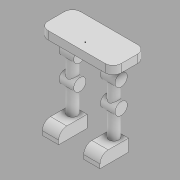
# Autodesk Inventor part: stick nodes
Saved by Autodesk Inventor 2021 (Build 250183000, 183)
## iProperties
Created: 2022-07-21
Part Number: stick nodes
Material: Generic
Document SubType Name: Modeling
Designer: Ahmed badghaish
Density: 1 g/cm^3
Appearance: Default
Author: Ahmed badghaish
Autodesk Inventor part; units mm, degrees
sketch "Sketch1" plane through (0, 0, 0) normal (0, 0, 1) x (1, 0, 0)
  line L0 (0, 0) -> (0, 200)
  line L1 (0, 0) -> (-50, 0)
  line L2 (0, 0) -> (50, 0)
  line L3 (-15.3846, 0) -> (-35.3846, 0)
  line L4 (-35.3846, 0) -> (-35.3846, 15)
  line L5 (-35.3846, 15) -> (-15.3846, 15)
  line L6 (-15.3846, 15) -> (-15.3846, 0)
  line L7 (35.3846, 0) -> (35.3846, 15)
  line L8 (35.3846, 15) -> (15.3846, 15)
  line L9 (15.3846, 15) -> (15.3846, 0)
  dimension "d0" = 200
  dimension "d1" = 0
  dimension "d2" = 50
  dimension "d3" = 50
  dimension "d4" = 20
  dimension "d5" = 15
  constraints: 20 end point, 4 symmetric about line, 2 horizontal, 2 parallel, 2 point on line, 1 perpendicular, 1 vertical
  measures "d0" distance of L0.start L0.end
  measures "d1" distance of point (0, 0) L0.start
  measures "d2" distance of L0.start L1.end
  measures "d3" distance of L0.start L2.end
  measures "d4" distance of L4.end L5.end
  measures "d5" distance of L3.end L4.end
extrude "Extrusion1" add sketch "Sketch1" along normal mid plane 35
fillet "Fillet1" radius 10 2 edges at (25.3846, 15, 17.5) (-25.3846, 15, 17.5)
sketch "Sketch2" plane through (-35.3846, 15, -17.5) normal (0, 1, 0) x (1, 0, 0)
  circle A0 centre (10, -8) radius 6
  line L0 (20, 0) -> (20, -25) projected
  line L1 (0, 0) -> (20, 0) projected
  circle A1 centre (60.7692, -8) radius 6
  line L2 (70.7692, 0) -> (70.7692, -25) projected
  line L3 (50.7692, 0) -> (70.7692, 0) projected
  point P0 (35.3846, -17.5)
  dimension "d9" = 12
  dimension "d10" = 10
  dimension "d11" = 8
  dimension "d12" = 12
  dimension "d13" = 10
  dimension "d14" = 8
  constraints: 2 centre point
  measures "d9" diameter of A0
  measures "d10" distance from line of L0 A0.centre
  measures "d11" distance from line of L1 A0.centre
  measures "d12" diameter of A1
  measures "d13" distance from line of L2 A1.centre
  measures "d14" distance from line of L3 A1.centre
extrude "Extrusion2" add sketch "Sketch2" along normal blind 35
ref_plane "Work Plane1" through (-25.3846, 0, -17.5) normal (1, 0, 0) x (0, 0, -1)
sketch "Sketch3" plane through (-25.3846, 0, -17.5) normal (1, 0, 0) x (0, 0, -1)
  line L0 (-2, 50) -> (-14, 50) projected
  circle A0 centre (-8, 50) radius 7.5
  point P0 (-17.5, 0)
  dimension "d17" = 15
  constraints: 1 centre point, 1 midpoint
  measures "d17" diameter of A0
extrude "Extrusion3" add sketch "Sketch3" along normal mid plane 18
ref_plane "Work Plane2" through (25.3846, 0, -17.5) normal (1, 0, 0) x (0, 0, -1)
sketch "Sketch4" plane through (25.3846, 0, -17.5) normal (1, 0, 0) x (0, 0, -1)
  line L0 (-2, 50) -> (-14, 50) projected
  circle A0 centre (-8, 50) radius 7.5
  point P0 (-17.5, 0)
  constraints: 1 centre point, 1 midpoint
extrude "Extrusion4" add sketch "Sketch4" along normal mid plane 18
ref_plane "Work Plane3" through (-35.3846, 57.5, -17.5) normal (0, 1, 0) x (1, 0, 0)
sketch "Sketch5" plane through (-35.3846, 57.5, -17.5) normal (0, 1, 0) x (1, 0, 0)
  circle A0 centre (10, -8) radius 6
  line L0 (20, 0) -> (20, -25) projected
  line L1 (0, 0) -> (20, 0) projected
  point P0 (35.3846, -17.5)
  dimension "d23" = 12
  dimension "d24" = 10
  dimension "d25" = 8
  constraints: 1 centre point
  measures "d23" diameter of A0
  measures "d24" distance from line of L0 A0.centre
  measures "d25" distance from line of L1 A0.centre
extrude "Extrusion5" add sketch "Sketch5" along normal blind 23 and the other way blind 3
ref_plane "Work Plane4" through (0, 0, -17.5) normal (-1, 0, 0) x (0, 0, 1)
mirror "Mirror1" about plane through (0, 0, -17.5) normal (-1, 0, 0) of "Extrusion3", "Extrusion5"
ref_plane "Work Plane5" through (-25.3846, 0, -17.5) normal (1, 0, 0) x (0, 0, -1)
sketch "Sketch6" plane through (-25.3846, 0, -17.5) normal (1, 0, 0) x (0, 0, -1)
  line L0 (-14, 80.5) -> (-2, 80.5) projected
  circle A0 centre (-8, 80.5) radius 7.5
  point P0 (-17.5, 0)
  dimension "d30" = 15
  constraints: 1 centre point, 1 midpoint
  measures "d30" diameter of A0
extrude "Extrusion6" add sketch "Sketch6" along normal mid plane 18
mirror "Mirror2" about plane through (0, 0, -17.5) normal (-1, 0, 0) of "Extrusion6"
ref_plane "Work Plane6" through (-25.3846, 88, -9.5) normal (0, 1, 0) x (-1, 0, 0)
sketch "Sketch7" plane through (-25.3846, 88, -9.5) normal (0, 1, 0) x (-1, 0, 0)
  circle A0 centre (0, 0) radius 6
  line L0 (-10, -8) -> (-10, 17) projected
  line L1 (10, -8) -> (-10, -8) projected
  point P0 (-25.3846, 9.5)
  dimension "d33" = 12
  dimension "d34" = 10
  dimension "d35" = 8
  constraints: 1 centre point
  measures "d33" diameter of A0
  measures "d34" distance from line of L0 A0.centre
  measures "d35" distance from line of L1 A0.centre
extrude "Extrusion7" add sketch "Sketch7" along normal blind 20 and the other way blind 3
ref_plane "Work Plane7" through (0, 0, -17.5) normal (-1, 0, 0) x (0, 0, 1)
mirror "Mirror3" about plane through (0, 0, -17.5) normal (-1, 0, 0) of "Extrusion7"
sketch "Sketch8" plane through (25.3846, 108, -9.5) normal (0, 1, 0) x (1, 0, 0)
  line L0 (19.2308, -20) -> (-70.7692, -20)
  line L1 (-70.7692, -20) -> (-70.7692, 20)
  line L2 (-70.7692, 20) -> (19.2308, 20)
  line L3 (19.2308, 20) -> (19.2308, -20)
  circle A0 centre (-50.7692, 0) radius 6 projected
  circle A1 centre (0, 0) radius 6 projected
  point P0 (-25.3846, -9.5)
  dimension "d40" = 90
  dimension "d41" = 40
  dimension "d42" = 20
  dimension "d43" = 20
  constraints: 8 end point, 2 parallel, 1 horizontal, 1 perpendicular
  measures "d40" distance of L1.end L2.end
  measures "d41" distance of L0.end L1.end
  measures "d42" distance from line of L1 A0.centre
  measures "d43" distance from line of A1.centre L2
extrude "Extrusion8" add sketch "Sketch8" against normal blind 10
sketch "Sketch9" plane through (-25.3846, 108, -9.5) normal (0, 1, 0) x (1, 0, 0)
  point P0 (25.3846, -9.5)
fillet "Fillet2" radius 10 4 edges at (-45.3846, 103, 10.5) (44.6154, 103, 10.5) (44.6154, 103, -29.5) (-45.3846, 103, -29.5)
body "Solid1"
